Faucet Hole (Autodesk Fusion 360 design; units mm, degrees)
Autodesk Fusion 360 part; units mm, degrees
sketch "Sketch1" plane through (0, 0, 0) normal (0, 0, 1) x (1, 0, 0)
  circle A0 centre (0, 0) radius 23
  circle A1 centre (0, 0) radius 14
  circle A2 centre (0, 0) radius 17
  dimension "d1" = 46
  dimension "d2" = 28
  dimension "d3" = 34
  constraint coincident A0.centre A1.centre
  constraint concentric A0 A2
  measures "d1" diameter of A0
  measures "d2" diameter of A1
  measures "d3" diameter of A2
extrude "Extrude1" add sketch "Sketch1" along normal blind 3 contours A0 | A2
extrude "Extrude2" add sketch "Sketch1" against normal blind 8 contours A2
